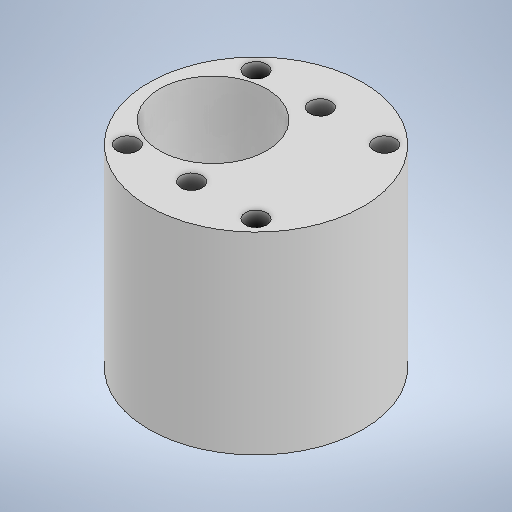
# Autodesk Inventor part: 11
Saved by Autodesk Inventor 2025.1 (Build 291241000, 241)
## iProperties
Created: 2024-09-17
Part Number: 11
Material: Generisch
Document SubType Name: Modeling
Designer: ffogue
Density: 1 g/cm^3
Appearance: Vorgabe
Author: ffogue
Autodesk Inventor part; units mm, degrees
ref_plane "YZ Plane" through (0, 0, 0) normal (1, 0, 0) x (0, 1, 0)
ref_plane "XZ Plane" through (0, 0, 0) normal (0, 1, 0) x (-1, 0, 0)
ref_plane "XY Plane" through (0, 0, 0) normal (0, 0, 1) x (1, 0, 0)
sketch "Sketch1" plane through (0, 0, 0) normal (0, 0, 1) x (1, 0, 0)
  circle A0 centre (0, 0) radius 10
  circle A1 centre (-6, 6) radius 1
  circle A2 centre (0, 6) radius 1
  circle A3 centre (6, 6) radius 1
  circle A4 centre (6, -6) radius 1
  circle A5 centre (0, -6) radius 1
  circle A6 centre (-6, -6) radius 1
  dimension "d0" = 20
  dimension "d2" = 2
  dimension "d3" = 12
  dimension "d4" = 6
  dimension "d5" = 12
  dimension "d6" = 6
  dimension "d7" = 6
  dimension "d8" = 2
  constraints: 7 centre point, 4 equal radius, 4 horizontal alignment, 4 vertical alignment, 1 coincident
  measures "d0" diameter of A0
  measures "d2" diameter of A6
  measures "d3" distance of A6.centre A1.centre
  measures "d4" horizontal distance of point (0, 0) A6.centre
  measures "d5" distance of A4.centre A6.centre
  measures "d6" horizontal distance of point (0, 0) A6.centre
  measures "d7" horizontal distance of point (0, 0) A1.centre
  measures "d8" diameter of A1
extrude "Extrusion1" add sketch "Sketch1" along normal blind 18
sketch "Sketch2" plane through (0, 0, 18) normal (0, 0, -1) x (-1, 0, 0)
  circle A0 centre (4, 0) radius 5
  circle A1 centre (0, 6) radius 1 projected
  point P0 (0, 0)
  dimension "d11" = 10
  dimension "d12" = 4
  constraints: 1 centre point, 1 horizontal alignment
  measures "d11" diameter of A0
  measures "d12" horizontal distance of A1.centre A0.centre
extrude "Extrusion2" cut sketch "Sketch2" along normal blind 18 contours A0
equation "\"d4\" = 0.5 * d3"
equation "\"d6\" = 0.5 * d5"
body "Solid1"
